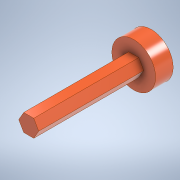
# Autodesk Inventor part: 1_2x3-inchHexShaft
Saved by Autodesk Inventor 2021.2 (Build 252289000, 289)
## iProperties
Created: 2020-11-16
Part Number: 1_2x3-inchHexShaft
Material: PC/ABS Plastic
Document SubType Name: Modeling
Designer: robst
Density: 0.357273 g/cm^3
Appearance: Smooth - Light Orange
Author: robst
Autodesk Inventor part; units mm, degrees
ref_plane "YZ Plane" through (0, 0, 0) normal (1, 0, 0) x (0, 1, 0)
ref_plane "XZ Plane" through (0, 0, 0) normal (0, 1, 0) x (-1, 0, 0)
ref_plane "XY Plane" through (0, 0, 0) normal (0, 0, 1) x (1, 0, 0)
sketch "Sketch1" plane through (0, 0, 0) normal (0, 0, 1) x (1, 0, 0)
  line L0 (7.259, 0) -> (3.6295, -6.2865)
  line L1 (3.6295, -6.2865) -> (-3.6295, -6.2865)
  line L2 (-3.6295, -6.2865) -> (-7.259, 0)
  line L3 (-7.259, 0) -> (-3.6295, 6.2865)
  line L4 (-3.6295, 6.2865) -> (3.6295, 6.2865)
  line L5 (3.6295, 6.2865) -> (7.259, 0)
  point P0 (0, 0)
  point P1 (0, 0)
  dimension "d0" = 12.573
  constraints: 12 end point, 1 coincident, 1 horizontal, 13 other
  measures "d0" distance between parallel lines of L1 L4
extrude "Extrusion1" add sketch "Sketch1" along normal mid plane 76.2
sketch "Sketch2" plane through (0, 0, -38.1) normal (0, 0, -1) x (-1, 0, 0)
  circle A0 centre (0, 0) radius 15.875
  dimension "d3" = 31.75
  constraints: 1 centre point, 1 coincident
  measures "d3" diameter of A0
extrude "Extrusion2" add sketch "Sketch2" along normal blind 12.7
equation "\"d0\" = printedHexSize"
equation "\"d1\" = length"
equation "\"hexSize\" = 12.7"
equation "\"slipFitOffset\" = 0.127"
equation "\"printedHexSize\" = hexSize - slipFitOffset"
equation "\"length\" = 76.2"
body "Solid1"
